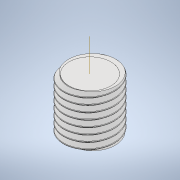
# Autodesk Inventor part: threadTeset
Saved by Autodesk Inventor 2022 (Build 260153000, 153)
## iProperties
Created: 2021-10-06
Part Number: threadTeset
Material: Generic
Document SubType Name: Modeling
Designer: tecware
Density: 1 g/cm^3
Appearance: Default
Author: tecware
Autodesk Inventor part; units mm, degrees
ref_plane "YZ Plane" through (0, 0, 0) normal (1, 0, 0) x (0, 1, 0)
ref_plane "XZ Plane" through (0, 0, 0) normal (0, 1, 0) x (-1, 0, 0)
ref_plane "XY Plane" through (0, 0, 0) normal (0, 0, 1) x (1, 0, 0)
sketch "Sketch3" plane through (0, 0, 0) normal (0, 0, 1) x (1, 0, 0)
  point P0 (0, 0)
sketch "Sketch4" plane through (0, 0, 0) normal (0, 1, 0) x (-1, 0, 0)
  circle A0 centre (0, 0) radius 10
  dimension "d7" = 20
  constraints: 1 centre point, 1 coincident
  measures "d7" diameter of A0
extrude "Extrusion2" add sketch "Sketch4" along normal blind 20
thread "Thread2" size "M20x2.5" class "6g" standard "ANSI Metric M Profile" full length
sketch "Sketch6" plane through (0, 20, 0) normal (1, 0, 0) x (0, 0, 1)
  line L0 (10, 0) -> (10, 20)
  line L1 (10, 20) -> (8.1463, 20)
  line L2 (8.1463, 20) -> (8.1463, 0)
  line L3 (8.1463, 0) -> (10, 0)
  line L4 (0, -7.2713) -> (0, 24.5452) projected
  constraints: 8 end point
revolve "Revolution1" cut sketch "Sketch6" angle 360 about axis through (0, 20, 0) along (0, -1, 0)
sketch "Sketch7" plane through (0, 20, 0) normal (1, 0, 0) x (0, 0, 1)
  line L0 (10, 0) -> (10, 20)
  line L1 (10, 20) -> (8.1463, 20)
  line L2 (8.1463, 20) -> (8.1463, 0)
  line L3 (8.1463, 0) -> (10, 0)
  line L4 (0, -7.2713) -> (0, 24.5452) projected
  constraints: 8 end point
revolve "Revolution2" add sketch "Sketch7" angle 360 about axis through (0, 20, 0) along (0, -1, 0) separate body
sketch "Sketch5" plane through (0, 20, 0) normal (-1, 0, 0) x (0, -1, 0)
  line L0 (-1.4584, -8.2729) -> (-1.2501, -8.2729) construction
  line L1 (0.2082, -9.8737) -> (-0.0001, -10.274) construction
  line L2 (-2.5001, -10.274) -> (-2.7084, -9.8737) construction
  line L3 (-1.0418, -8.2729) -> (-1.2501, -7.8727) construction
  line L4 (-1.2501, -7.8727) -> (-1.4584, -8.2729) construction
  line L5 (-2.5001, -10.274) -> (-2.2918, -9.8737) construction
  line L6 (-1.0418, -8.2729) -> (-0.2084, -9.8737)
  line L7 (-2.7084, -9.8737) -> (-2.2918, -9.8737) construction
  arc A0 (-2.7084, -9.8737) -> (-2.5001, -10.0002) centre (-2.5001, -9.7653) ccw construction
  line L8 (0.2082, -9.8737) -> (-0.2084, -9.8737) construction
  line L9 (-2.5001, -10.274) -> (-2.5001, -9.8737) construction
  line L10 (-0.0001, -10.274) -> (-0.0001, -9.8737) construction
  line L11 (-1.2501, -7.8727) -> (-1.2501, -8.1465) construction
  line L12 (-2.5001, -10.0002) -> (-0.0001, -10.0002)
  arc A1 (-2.5001, -10.0002) -> (-2.2918, -9.8737) centre (-2.5001, -9.7653) ccw
  line L13 (-0.2084, -9.8737) -> (-0.0001, -10.274) construction
  line L14 (-2.2918, -9.8737) -> (-1.4584, -8.2729)
  line L15 (-0.0001, -0.0002) -> (-0.0001, 0.0177)
  line L16 (-0.0001, 0.0177) -> (-0.0001, -0.0002)
  line L17 (-0.0001, -0.0002) -> (0.0334, -0.0002)
  arc A2 (-0.2084, -9.8737) -> (-0.0001, -10.0002) centre (-0.0001, -9.7653) ccw
  arc A3 (-0.0001, -10.0002) -> (0.2082, -9.8737) centre (-0.0001, -9.7653) ccw construction
  arc A4 (-1.2501, -8.1465) -> (-1.4584, -8.2729) centre (-1.2501, -8.3814) ccw
  arc A5 (-1.0418, -8.2729) -> (-1.2501, -8.1465) centre (-1.2501, -8.3814) ccw
  line L18 (-1.2501, -8.1465) -> (-1.2501, -8.2729) construction
  line L19 (-1.2501, -8.2729) -> (-1.0418, -8.2729) construction
  dimension "d10" = 55
  dimension "d11" = 0.4002
  dimension "d12" = 0.4002
  dimension "Sketch5_ThreadOffset" = 0
  dimension "Sketch5_MajorRadius" = 10
  dimension "d15" = 2.5
  dimension "Sketch5_MinorRadius" = 8.1463
  constraints: 40 end point, 12 point on circle, 10 parallel, 8 tangent, 6 centre point, 6 collinear, 2 midpoint, 2 point on line, 1 horizontal, 1 perpendicular, 3 other
  measures "d10" angle of L6 L14
  measures "d11" distance of L3.end L0.end
  measures "d12" distance of L1.end L10.end
  measures "Sketch5_ThreadOffset" distance between parallel lines of L15 L10
  measures "Sketch5_MajorRadius" distance from line of L12 L15.start
  measures "d15" distance from line of L1.end L9
  measures "Sketch5_MinorRadius" distance edge to line of A5 L17
coil "Coil1" sketch "Sketch5" operation cut axis through (0, 20, 0) along (0, -1, 0) pitch 2.5025 turns 9.99001 hand right bodies 2
equation "\"d10\" = d17"
equation "\"d11\" = 0.160083 * Sketch5_Pitch"
equation "\"d12\" = 0.160083 * Sketch5_Pitch"
equation "\"d15\" = Sketch5_Pitch"
equation "\"d17\" = 55deg"
equation "\"Sketch5_Pitch\" = 2.5"
body "Solid2"
body "Solid3"
